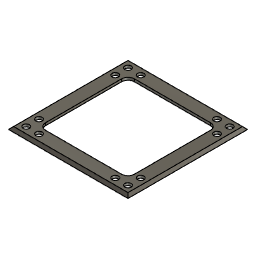
Frame base_lid v1 (Autodesk Fusion 360 design; units mm, degrees)
Autodesk Fusion 360 part; units mm, degrees
note: some values were not read from the file. Set by a fixed rule: which sketch regions a step uses.
sketch "Sketch1" plane through (0, 0, 0) normal (0, 0, 1) x (1, 0, 0)
  line L0 (0, 0) -> (100, 0)
  line L1 (100, 0) -> (100, 100)
  line L2 (100, 100) -> (0, 100)
  line L3 (0, 100) -> (0, 0)
  line L4 (0, 0) -> (15, 0)
  line L5 (15, 0) -> (15, 15)
  line L6 (100, 100) -> (85, 100)
  line L7 (85, 100) -> (85, 85)
  line L8 (15, 15) -> (85, 15)
  line L9 (85, 15) -> (85, 85)
  line L10 (85, 85) -> (15, 85)
  line L11 (15, 85) -> (15, 15)
  dimension "d1" = 100
  dimension "d2" = 100
  dimension "d3" = 15
  dimension "d4" = 15
  dimension "d5" = 15
  dimension "d6" = 15
  constraint horizontal L0
  constraint vertical L1
  constraint horizontal L2
  constraint vertical L3
  constraint coincident L0.start L3.end
  constraint perpendicular L3 L4
  constraint perpendicular L0 L5
  constraint perpendicular L1 L6
  constraint perpendicular L2 L7
  constraint horizontal L8
  constraint vertical L9
  constraint horizontal L10
  constraint vertical L11
  measures "d1" distance of L0.start L0.end
  measures "d2" distance of L0.start L2.end
  measures "d3" distance of L0.start L4.end
  measures "d4" distance of L4.end L5.end
  measures "d5" distance of L1.end L6.end
  measures "d6" distance of L6.end L7.end
extrude "Extrude1" add sketch "Sketch1" along normal blind 5 contours L0 L2 L3 L4 L5 L7 L10 L11 | L0 L1 L2 L5 L6 L7 L8 L9
chamfer "Chamfer1" distance 5 angle 45 1 edges at (50, 0, 5)
chamfer "Chamfer2" distance 5 angle 45 1 edges at (0, 52.5, 5)
chamfer "Chamfer3" distance 5 angle 45 1 edges at (52.5, 100, 5)
chamfer "Chamfer4" distance 5 angle 45 1 edges at (100, 50, 5)
extrude "Extrude2" cut 1 faces at (5, 61.6667, 0) along direction (0, 0, 1) blind 3
sketch "Sketch2" plane through (0, 0, 5) normal (0, 0, 1) x (-1, 0, 0)
  line L0 (-15, -15) -> (-15, -85)
  line L1 (-15, -85) -> (-85, -85)
  line L2 (-85, -85) -> (-85, -15)
  line L3 (-85, -15) -> (-15, -15)
  line L4 (-95, -5) -> (-95, -95)
  line L5 (-95, -95) -> (-5, -95)
  line L6 (-5, -95) -> (-5, -5)
  line L7 (-5, -5) -> (-95, -5)
  circle A0 centre (-10, -90) radius 2.5
  line L8 (-10, -90) -> (-20, -90)
  circle A1 centre (-20, -90) radius 2.5
  line L9 (-10, -90) -> (-10, -80)
  circle A2 centre (-10, -80) radius 2.5
  circle A3 centre (-90, -90) radius 2.5
  line L10 (-90, -90) -> (-90, -80)
  line L11 (-90, -90) -> (-80, -90)
  circle A4 centre (-90, -80) radius 2.5
  circle A5 centre (-80, -90) radius 2.5
  circle A6 centre (-90, -10) radius 2.5
  line L12 (-90, -10) -> (-90, -20)
  line L13 (-90, -10) -> (-80, -10)
  circle A7 centre (-80, -10) radius 2.5
  circle A8 centre (-90, -20) radius 2.5
  circle A9 centre (-10, -10) radius 2.5
  line L14 (-10, -10) -> (-20, -10)
  line L15 (-10, -10) -> (-10, -20)
  circle A10 centre (-20, -10) radius 2.5
  circle A11 centre (-10, -20) radius 2.5
  dimension "d15" = 5
  dimension "d16" = 10
  dimension "d17" = 5
  dimension "d18" = 10
  dimension "d19" = 5
  dimension "d20" = 5
  dimension "d21" = 10
  dimension "d22" = 10
  dimension "d23" = 5
  dimension "d24" = 5
  dimension "d25" = 5
  dimension "d26" = 10
  dimension "d27" = 10
  dimension "d28" = 5
  dimension "d29" = 5
  dimension "d30" = 5
  dimension "d31" = 10
  dimension "d32" = 10
  dimension "d33" = 5
  dimension "d34" = 5
  constraint coincident A0.centre L8.start
  constraint horizontal L8
  constraint coincident L8.end A1.centre
  constraint perpendicular L8 L9
  constraint coincident L9.end A2.centre
  constraint coincident A3.centre L10.start
  constraint parallel L4 L10
  constraint perpendicular L10 L11
  constraint coincident L10.end A4.centre
  constraint coincident L11.end A5.centre
  constraint coincident A6.centre L12.start
  constraint vertical L12
  constraint perpendicular L12 L13
  constraint coincident L13.end A7.centre
  constraint coincident L12.end A8.centre
  constraint coincident A9.centre L14.start
  constraint horizontal L14
  constraint perpendicular L14 L15
  constraint coincident L14.end A10.centre
  constraint coincident L15.end A11.centre
  measures "d15" diameter of A0
  measures "d16" distance of A0.centre L8.end
  measures "d17" diameter of A1
  measures "d18" distance of A0.centre L9.end
  measures "d19" diameter of A2
  measures "d20" diameter of A3
  measures "d21" distance of A3.centre L10.end
  measures "d22" distance of A3.centre L11.end
  measures "d23" diameter of A4
  measures "d24" diameter of A5
  measures "d25" diameter of A6
  measures "d26" distance of A6.centre L12.end
  measures "d27" distance of A6.centre L13.end
  measures "d28" diameter of A7
  measures "d29" diameter of A8
  measures "d30" diameter of A9
  measures "d31" distance of A9.centre L14.end
  measures "d32" distance of A9.centre L15.end
  measures "d33" diameter of A10
  measures "d34" diameter of A11
extrude "Extrude3" cut sketch "Sketch2" against normal blind 5 contours A0 L8 L9 | A0 L8 L9 | A1 | A2 | A3 L10 L11 | A3 L10 L11 | A4 | A5 | A6 L12 L13 | A6 L12 L13 | A7 | A8 | A9 L14 L15 | A9 L14 L15 | A10 | A11
fillet "Fillet1" radius 5 1 edges at (15, 85, 4)
fillet "Fillet2" radius 5 1 edges at (85, 15, 4)
fillet "Fillet3" radius 5 1 edges at (15, 15, 4)
fillet "Fillet4" radius 5 1 edges at (85, 85, 4)
